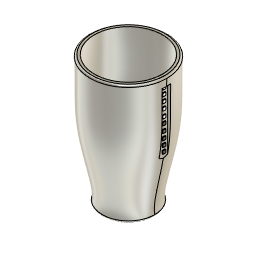
MoneyMug v4 (Autodesk Fusion 360 design; units mm, degrees)
Autodesk Fusion 360 part; units mm, degrees
sketch "Sketch3" plane through (0, 0, 95) normal (0, 0, 1) x (-1, 0, 0)
sketch "Sketch4" plane through (0, 0, 0) normal (0, 1, 0) x (1, 0, 0)
  line L0 (0, 0) -> (0.5, 0)
  line L1 (0, 0) -> (0.5, 0)
  line L2 (0.5, 0) -> (28.5799, 0)
  line L3 (0, 0) -> (0, -5)
  line L4 (40, -150) -> (42.7494, -150)
  spline S0 degree 5 poles (30.8084, -2.5598) (30.7478, -2.9959) (30.6285, -3.9398) (30.4557, -5.5709) (30.3036, -8.2723) (30.5448, -12.9536) (31.4015, -19.166) (32.8511, -26.8019) (34.7518, -35.5621) (36.8814, -45.0209) (38.9948, -54.7224) (40.8692, -64.2541) (42.3643, -73.3472) (43.4405, -81.906) (44.1249, -89.9512) (44.4922, -97.5873) (44.6403, -104.9616) (44.6707, -112.2309) (44.6634, -119.519) (44.6686, -126.9023) (44.7162, -134.4257) (44.7995, -140.5726) (44.8892, -145.2574) (44.961, -148.4136) (45, -150) knots 0 0 0 0 0 0 0.05 0.1 0.15 0.2 0.25 0.3 0.35 0.4 0.45 0.5 0.55 0.6 0.65 0.7 0.75 0.8 0.85 0.9 0.95 1 1 1 1 1 1
  arc A0 (30.8084, -2.5598) -> (28.5799, 0) centre (28.5799, -2.25) ccw
  arc A1 (42.7494, -150) -> (44.9994, -147.7487) centre (42.7494, -147.75) ccw
  spline S1 degree 5 poles (40, -150) (39.9691, -148.501) (39.9142, -145.5203) (39.8524, -141.1017) (39.8114, -135.3152) (39.8247, -128.2509) (39.8886, -121.3344) (39.9738, -114.5205) (40.0311, -107.7329) (39.9838, -100.8514) (39.73, -93.7161) (39.1684, -86.1672) (38.219, -78.0782) (36.8458, -69.3912) (35.0797, -60.1525) (33.0415, -50.5496) (30.9671, -40.9495) (29.1344, -31.818) (27.7899, -23.6388) (27.0781, -16.8345) (26.9608, -11.6805) (27.1569, -8.2352) (27.0241, -6.2194) (25.7395, -5.1513) (22.6987, -4.6554) (17.5738, -4.5184) (11.682, -4.6061) (6.2386, -4.7665) (2.1552, -4.9152) (0, -5) knots 0 0 0 0 0 0 0.04 0.08 0.12 0.16 0.2 0.24 0.28 0.32 0.36 0.4 0.44 0.48 0.52 0.56 0.6 0.64 0.68 0.72 0.76 0.8 0.84 0.88 0.92 0.96 1 1 1 1 1 1
  point P0 (30.5, 0)
  point P1 (30.5, -10.9625)
  point P2 (40, -60)
  point P3 (44.6467, -108.7425)
  point P4 (40, -110)
  point P5 (35, -60)
  point P6 (27.0469, -10.7982)
  point P7 (26.3491, -5.9135)
  dimension "d9" = 30
  dimension "d12" = 2.25
  constraint coincident L0.start L1.start
  constraint horizontal L0
  constraint horizontal L1
  constraint parallel L0 L2
  constraint perpendicular L2 L3
  constraint perpendicular L3 L4
  constraint coincident P0 L2
  constraint tangent L2 A0
  constraint tangent S0 A0
  constraint coincident S0.end L4
  constraint tangent L4 A1
  constraint tangent S0 A1
  constraint equal A0 A1
  measures "d9" distance of L0.end P0
  measures "d12" radius of A0
revolve "Revolve1" add sketch "Sketch4" angle 360 about axis through (0, 0, 1.75) along (0, 0, 1) makes body 1
sketch "Sketch5" plane through (0, 0, 0) normal (1, 0, 0) x (0, 1, 0)
  line L0 (-5, 140) -> (5, 140)
  line L1 (5, 140) -> (5, 60)
  line L2 (-5, 60) -> (-5, 140)
  dimension "d14" = 80
  dimension "d15" = 10
  constraint horizontal L0
  constraint vertical L1
  constraint vertical L2
  measures "d14" distance of L0.start L2.start
  measures "d15" distance of L0.start L0.end
sketch "Sketch6" plane through (0, 0, 100) normal (1, 0, 0) x (0, 1, 0)
  line L0 (-5, 40) -> (5, 40)
  line L1 (5, 40) -> (5, -40)
  line L2 (5, -40) -> (-5, -40)
  line L3 (-5, -40) -> (-5, 40)
  constraint horizontal L0
  constraint vertical L1
  constraint horizontal L2
  constraint vertical L3
extrude "Extrude3" cut sketch "Sketch6" along normal blind 41 and the other way blind -45 bodies 1
sketch "Sketch7" plane through (41, 0, 0) normal (1, 0, 0) x (0, 1, 0)
  spline S0 degree 3 poles (0, 65.407) (-0.0911, 65.407) (-0.1824, 65.4087) (-1.0234, 65.4406) (-1.7546, 65.5851) (-3.3709, 66.1404) (-4.2183, 66.6057) (-5, 67.1629) knots -0.602881 -0.602881 -0.602881 -0.602881 -0.57542 -0.57542 -0.350239 -0.350239 -0.0625 -0.0625 -0.0625 -0.0625
  spline S1 degree 3 poles (5, 67.1629) (4.8291, 67.0411) (4.655, 66.9236) (3.659, 66.2916) (2.776, 65.8808) (1.2329, 65.4869) (0.6202, 65.407) (0, 65.407) knots -1.14383 -1.14383 -1.14383 -1.14383 -1.080888 -1.080888 -0.789829 -0.789829 -0.602881 -0.602881 -0.602881 -0.602881
  line L0 (5, 67.1629) -> (5, 140)
  line L1 (5, 140) -> (-5, 140)
  line L2 (-5, 140) -> (-5, 67.1629)
  line L3 (-1.5344, 138.974) -> (1.9665, 138.974)
  line L4 (1.9665, 138.974) -> (1.9665, 135.4732)
  line L5 (1.9665, 135.4732) -> (-1.5344, 135.4732)
  line L6 (-1.5344, 135.4732) -> (-1.5344, 138.974)
  line L7 (-1.5344, 131.9658) -> (1.9665, 131.9658)
  line L8 (1.9665, 131.9658) -> (1.9665, 128.4649)
  line L9 (1.9665, 128.4649) -> (-1.5344, 128.4649)
  line L10 (-1.5344, 128.4649) -> (-1.5344, 131.9658)
  line L11 (-1.5344, 124.8596) -> (1.9665, 124.8596)
  line L12 (1.9665, 124.8596) -> (1.9665, 121.3588)
  line L13 (1.9665, 121.3588) -> (-1.5344, 121.3588)
  line L14 (-1.5344, 121.3588) -> (-1.5344, 124.8596)
  line L15 (-1.5344, 117.4414) -> (1.9665, 117.4414)
  line L16 (1.9665, 117.4414) -> (1.9665, 113.9405)
  line L17 (1.9665, 113.9405) -> (-1.5344, 113.9405)
  line L18 (-1.5344, 113.9405) -> (-1.5344, 117.4414)
  line L19 (-1.5344, 109.4567) -> (1.9665, 109.4567)
  line L20 (1.9665, 109.4567) -> (1.9665, 105.9559)
  line L21 (1.9665, 105.9559) -> (-1.5344, 105.9559)
  line L22 (-1.5344, 105.9559) -> (-1.5344, 109.4567)
  line L23 (-1.5344, 102.4622) -> (1.9665, 102.4622)
  line L24 (1.9665, 102.4622) -> (1.9665, 98.9613)
  line L25 (1.9665, 98.9613) -> (-1.5344, 98.9613)
  line L26 (-1.5344, 98.9613) -> (-1.5344, 102.4622)
  line L27 (-1.5344, 94.7328) -> (1.9665, 94.7328)
  line L28 (1.9665, 94.7328) -> (1.9665, 91.232)
  line L29 (1.9665, 91.232) -> (-1.5344, 91.232)
  line L30 (-1.5344, 91.232) -> (-1.5344, 94.7328)
  line L31 (-1.5344, 87.2753) -> (1.9665, 87.2753)
  line L32 (1.9665, 87.2753) -> (1.9665, 83.7744)
  line L33 (1.9665, 83.7744) -> (-1.5344, 83.7744)
  line L34 (-1.5344, 83.7744) -> (-1.5344, 87.2753)
  line L35 (-1.5344, 80.5033) -> (1.9665, 80.5033)
  line L36 (1.9665, 80.5033) -> (1.9665, 77.0024)
  line L37 (1.9665, 77.0024) -> (-1.5344, 77.0024)
  line L38 (-1.5344, 77.0024) -> (-1.5344, 80.5033)
  line L39 (-1.5344, 73.6031) -> (1.9665, 73.6031)
  line L40 (1.9665, 73.6031) -> (1.9665, 70.1022)
  line L41 (1.9665, 70.1022) -> (-1.5344, 70.1022)
  line L42 (-1.5344, 70.1022) -> (-1.5344, 73.6031)
  constraint horizontal L3
  constraint vertical L4
  constraint horizontal L5
  constraint vertical L6
  constraint horizontal L7
  constraint vertical L8
  constraint horizontal L9
  constraint vertical L10
  constraint horizontal L11
  constraint vertical L12
  constraint horizontal L13
  constraint vertical L14
  constraint horizontal L15
  constraint vertical L16
  constraint horizontal L17
  constraint vertical L18
  constraint horizontal L19
  constraint vertical L20
  constraint horizontal L21
  constraint vertical L22
  constraint horizontal L23
  constraint vertical L24
  constraint horizontal L25
  constraint vertical L26
  constraint horizontal L27
  constraint vertical L28
  constraint horizontal L29
  constraint vertical L30
  constraint horizontal L31
  constraint vertical L32
  constraint horizontal L33
  constraint vertical L34
  constraint horizontal L35
  constraint vertical L36
  constraint horizontal L37
  constraint vertical L38
  constraint horizontal L39
  constraint vertical L40
  constraint horizontal L41
  constraint vertical L42
  constraint equal L4 L8
  constraint equal L8 L12
  constraint equal L12 L16
  constraint equal L16 L20
  constraint equal L20 L24
  constraint equal L24 L28
  constraint equal L28 L32
  constraint equal L32 L36
  constraint equal L36 L40
  constraint equal L35 L39
  constraint equal L31 L35
  constraint equal L27 L31
  constraint equal L23 L27
  constraint equal L19 L23
  constraint equal L15 L19
  constraint equal L11 L15
  constraint equal L7 L11
  constraint equal L3 L7
  constraint equal L31 L32
  constraint collinear L4 L8
  constraint collinear L8 L12
  constraint collinear L12 L16
  constraint collinear L16 L20
  constraint collinear L20 L24
  constraint collinear L24 L28
  constraint collinear L28 L32
  constraint collinear L32 L36
  constraint collinear L36 L40
extrude "Extrude4" add sketch "Sketch7" along normal blind 1 separate body contours L3 L4 L5 L6 | L7 L8 L9 L10 | L11 L12 L13 L14 | L15 L16 L17 L18 | L19 L20 L21 L22 | L23 L24 L25 L26 | L27 L28 L29 L30 | L31 L32 L33 L34 | L35 L36 L37 L38 | L39 L40 L41 L42 makes body 2 at (41, -0.3674, 86.1083) makes body 3 at (41, 0.7995, 115.1075) makes body 4 at (41, -0.3674, 136.6401) makes body 5 at (41, -0.3674, 108.2898) makes body 6 at (41, -0.3674, 79.3363) makes body 7 at (41, -0.3674, 93.5659) makes body 8 at (41, 0.7995, 122.5257) makes body 9 at (41, -0.3674, 130.7988) makes body 10 at (41, 0.7995, 100.1283) makes body 11 at (41, -0.3674, 72.4361)
sketch "Sketch8" plane through (0, 0, 0) normal (1, 0, 0) x (0, 1, 0)
sketch "Sketch9" plane through (0, 0, 0) normal (1, 0, 0) x (0, 1, 0)
sketch "Sketch10" plane through (0, 0, 0) normal (0, 0, 1) x (1, 0, 0)
  line L0 (-7.4201, 7.2472) -> (7.7528, 7.2472)
  line L1 (7.7528, 7.2472) -> (7.7528, -7.7528)
  line L2 (7.7528, -7.7528) -> (-7.4201, -7.7528)
  line L3 (-7.4201, -7.7528) -> (-7.4201, 7.2472)
  constraint horizontal L0
  constraint vertical L1
  constraint horizontal L2
  constraint vertical L3
extrude "Extrude5" cut sketch "Sketch10" along normal blind 2 bodies 11 10 9 8 7 6 5 4 3 2 1
sketch "Sketch11" plane through (0, 0, 0) normal (1, 0, 0) x (0, 1, 0)
  circle A0 centre (0, 125) radius 3.6887
extrude "Extrude6" add sketch "Sketch11" along normal blind -41 and the other way blind 46 separate body makes body 12
named bodies: "Mug", "LED8", "LED4", "LED1", "LED5", "LED9", "LED7", "LED3", "LED2", "LED6", "LED10", "Button"
